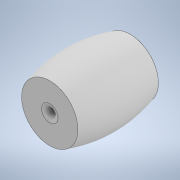
# Autodesk Inventor part: 5wheelroller
Saved by Autodesk Inventor 2021 (Build 250183000, 183)
## iProperties
Created: 2023-10-07
Part Number: 5wheelroller
Material: Generic
Document SubType Name: Modeling
Designer: Trey Vokoun
Density: 1 g/cm^3
Appearance: Default
Author: Trey Vokoun
Autodesk Inventor part; units mm, degrees
ref_plane "YZ Plane" through (0, 0, 0) normal (1, 0, 0) x (0, 1, 0)
ref_plane "XZ Plane" through (0, 0, 0) normal (0, 1, 0) x (-1, 0, 0)
ref_plane "XY Plane" through (0, 0, 0) normal (0, 0, 1) x (1, 0, 0)
sketch "Sketch1" plane through (0, 0, 0) normal (0, 1, 0) x (-1, 0, 0)
  line L0 (0, 0) -> (5.25, 0)
  line L1 (5.25, 0) -> (5.25, -15) construction
  line L2 (5.25, -15) -> (0, -15)
  line L3 (0, -15) -> (0, 0)
  arc A0 (5.25, -15) -> (5.25, 0) centre (-18.5985, -7.5) ccw
  line L4 (0.55, 0) -> (0.55, -15)
  dimension "d0" = 15
  dimension "d1" = 5.25
  dimension "d2" = 25
  dimension "d3" = 0.55
  constraints: 10 end point, 2 parallel, 2 perpendicular, 2 point on circle, 2 point on line, 1 centre point, 1 horizontal
  measures "d0" distance between parallel lines of L0 L2
  measures "d1" distance of L1.end L2.end
  measures "d2" radius of A0
  measures "d3" distance between parallel lines of L3 L4
revolve "Revolution1" add sketch "Sketch1" angle 360 about axis through (0, 0, -15) along (0, 0, 1) contours L0 A0 L2 L4
fillet "Fillet1" radius 1 2 edges at (0.55, 0, 0) (0.55, 0, -15)
body "Solid1"
